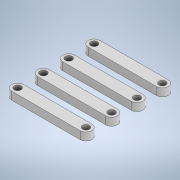
# Autodesk Inventor part: GARRA-palos
Saved by Autodesk Inventor 2021 (Build 250183000, 183)
## iProperties
Created: 2023-09-04
Part Number: GARRA-palos
Material: Generic
Document SubType Name: Modeling
Designer: PC
Density: 1 g/cm^3
Appearance: Default
Author: PC
Autodesk Inventor part; units mm, degrees
ref_plane "YZ Plane" through (0, 0, 0) normal (1, 0, 0) x (0, 1, 0)
ref_plane "XZ Plane" through (0, 0, 0) normal (0, 1, 0) x (-1, 0, 0)
ref_plane "XY Plane" through (0, 0, 0) normal (0, 0, 1) x (1, 0, 0)
sketch "Sketch1" plane through (0, 0, 0) normal (0, 1, 0) x (-1, 0, 0)
  circle A0 centre (0, 0) radius 1.75
  circle A1 centre (0, 0) radius 3
  line L0 (0, 0) -> (35, 0)
  circle A2 centre (35, 0) radius 1.75
  circle A3 centre (35, 0) radius 3
  line L1 (35, 3) -> (0, 3)
  line L2 (35, -3) -> (0, -3)
  dimension "d0" = 3.5
  dimension "d1" = 6
  dimension "d2" = 35
  dimension "d3" = 3.5
  dimension "d4" = 6
  constraints: 6 end point, 4 centre point, 4 coincident, 4 point on circle, 3 tangent, 1 horizontal
  measures "d0" diameter of A0
  measures "d1" diameter of A1
  measures "d2" distance of L0.start L0.end
  measures "d3" diameter of A2
  measures "d4" diameter of A3
extrude "Extrusion1" add sketch "Sketch1" along normal blind 4
sketch "Sketch2" plane through (0, 4, 0) normal (0, 1, 0) x (1, 0, 0)
  circle A0 centre (0, 13.1627) radius 3
  circle A1 centre (0, 13.1627) radius 1.75
  circle A2 centre (-35, 13.1627) radius 1.75
  circle A3 centre (-35, 13.1627) radius 3
  line L0 (-35, 16.1627) -> (0, 16.1627)
  line L1 (-35, 10.1627) -> (0, 10.1627)
  point P0 (0, 0)
  dimension "d7" = 6
  dimension "d8" = 3.5
  dimension "d9" = 3.5
  dimension "d10" = 6
  constraints: 4 centre point, 4 end point, 4 point on circle, 4 tangent, 2 coincident
  measures "d7" diameter of A0
  measures "d8" diameter of A1
  measures "d9" diameter of A2
  measures "d10" diameter of A3
extrude "Extrusion2" add sketch "Sketch2" against normal blind 4
sketch "Sketch3" plane through (0, 0, 0) normal (0, -1, 0) x (1, 0, 0)
  point P0 (0, 0)
sketch "Sketch4" plane through (0, 4, 0) normal (0, 1, 0) x (1, 0, 0)
  circle A0 centre (-35, 13.1627) radius 1.75 projected
  line L0 (-35, 13.1627) -> (-35, 26.1627)
  circle A1 centre (-35, 26.1627) radius 1.75
  circle A2 centre (-35, 26.1627) radius 3
  circle A3 centre (0, 26.1627) radius 1.75
  circle A4 centre (0, 26.1627) radius 3
  line L1 (-35, 29.1627) -> (0, 29.1627)
  line L2 (-35, 23.1627) -> (0, 23.1627)
  point P0 (0, 0)
  dimension "d13" = 13
  dimension "d14" = 3.5
  dimension "d15" = 6
  dimension "d16" = 3.5
  dimension "d17" = 6
  constraints: 6 end point, 4 centre point, 4 point on circle, 3 coincident, 2 tangent, 1 horizontal, 1 point on line, 1 vertical
  measures "d13" distance of L0.start L0.end
  measures "d14" diameter of A1
  measures "d15" diameter of A2
  measures "d16" diameter of A3
  measures "d17" diameter of A4
extrude "Extrusion3" add sketch "Sketch4" against normal blind 4 contours A2 | A2 L1 A4 L2 | A4
sketch "Sketch5" plane through (0, 4, 0) normal (0, 1, 0) x (1, 0, 0)
  circle A0 centre (-35, 26.1627) radius 1.75 projected
  line L0 (-35, 26.1627) -> (-35, 39.1627)
  circle A1 centre (-35, 39.1627) radius 3
  circle A2 centre (-35, 39.1627) radius 1.75
  circle A3 centre (0, 39.1627) radius 3
  circle A4 centre (0, 39.1627) radius 1.75
  line L1 (-35, 42.1627) -> (0, 42.1627)
  line L2 (0, 36.1627) -> (-35, 36.1627)
  point P0 (0, 0)
  dimension "d20" = 13
  dimension "d21" = 6
  dimension "d22" = 3.5
  dimension "d23" = 6
  dimension "d24" = 3.5
  constraints: 6 end point, 4 centre point, 4 point on circle, 3 coincident, 1 point on line, 1 tangent, 1 vertical
  measures "d20" distance of L0.start L0.end
  measures "d21" diameter of A1
  measures "d22" diameter of A2
  measures "d23" diameter of A3
  measures "d24" diameter of A4
extrude "Extrusion4" add sketch "Sketch5" against normal blind 4 contours A1 | A1 L1 A3 L2 | A3
sketch "Sketch6" plane through (0, 4, 0) normal (0, 1, 0) x (1, 0, 0)
  point P0 (0, 0)
body "Solid1"
